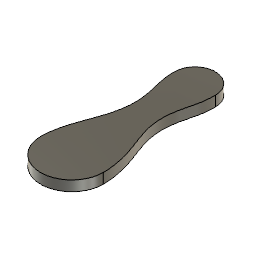
Linker (Autodesk Fusion 360 design; units mm, degrees)
part number: 2026-08-19-17-32-45-715
Autodesk Fusion 360 part; units mm, degrees
sketch "Sketch1" plane through (0, 0, 0) normal (0, 0, 1) x (1, 0, 0)
  circle A0 centre (0, 0) radius 30.539
  line L0 (0, 0) -> (0, 120)
  circle A1 centre (0, 120) radius 20
  spline S0 degree 5 poles (-20, 120) (-20, 118.6277) (-19.9377, 115.9337) (-19.6572, 112.0444) (-18.9403, 107.1368) (-17.656, 101.3217) (-16.2249, 95.6467) (-14.9004, 89.9411) (-13.9014, 84.0874) (-13.366, 78.0653) (-13.3647, 71.9193) (-13.9112, 65.7277) (-14.9727, 59.5726) (-16.479, 53.5086) (-18.3305, 47.5345) (-20.4074, 41.616) (-22.5782, 35.7039) (-24.7076, 29.7542) (-26.6645, 23.7473) (-28.3301, 17.7088) (-29.6027, 11.6919) (-30.2422, 6.9451) (-30.485, 3.446) (-30.539, 1.1436) (-30.539, 0) knots 0 0 0 0 0 0 0.05 0.1 0.15 0.2 0.25 0.3 0.35 0.4 0.45 0.5 0.55 0.6 0.65 0.7 0.75 0.8 0.85 0.9 0.95 1 1 1 1 1 1
  spline S1 degree 5 poles (30.539, 0) (30.539, 1.0785) (30.4943, 3.2756) (30.2934, 6.6915) (29.7578, 11.4626) (28.6529, 17.655) (27.1407, 23.9143) (25.276, 30.0944) (23.1495, 36.1084) (20.8974, 41.9731) (18.682, 47.7676) (16.6729, 53.5953) (15.0282, 59.5445) (13.8753, 65.6511) (13.2908, 71.8554) (13.2981, 78.0447) (13.8651, 84.101) (14.9009, 89.9465) (16.2511, 95.5906) (17.6914, 101.1783) (18.9706, 106.9311) (19.6763, 111.8544) (19.9473, 115.8136) (20.0032, 118.5829) (20, 120) knots 0 0 0 0 0 0 0.05 0.1 0.15 0.2 0.25 0.3 0.35 0.4 0.45 0.5 0.55 0.6 0.65 0.7 0.75 0.8 0.85 0.9 0.95 1 1 1 1 1 1
  line L1 (30.539, -11) -> (30.539, 11)
  line L2 (-30.539, 11.7182) -> (-30.539, -11.7182)
  line L3 (-20, 134) -> (-20, 106)
  line L4 (20.0327, 105.5399) -> (19.9673, 134.4601)
  point P0 (-30.539, 0)
  point P1 (30.539, 0)
  point P2 (-20, 120)
  point P3 (20, 120)
  point P4 (-24.7648, 29.445)
  point P5 (-15, 60)
  point P6 (-15, 90)
  point P7 (25.2479, 29.94)
  point P8 (15.0558, 60)
  point P9 (15, 90)
  point P10 (-15, 90)
  point P11 (-15, 60)
  point P12 (-24.7648, 29.445)
  point P13 (25.2479, 29.94)
  point P14 (15.0558, 60)
  point P15 (15, 90)
  dimension "d1" = 61.078
  dimension "d2" = 120
  dimension "d3" = 40
  constraint coincident A0.centre L0.start
  constraint vertical L0
  constraint coincident L0.end A1.centre
  constraint coincident A0 P0
  constraint coincident A0 P1
  constraint coincident A1 P2
  constraint coincident A1 P3
  constraint coincident P2 S0.start
  constraint coincident P10 P6
  constraint coincident P11 P5
  constraint coincident P12 P4
  constraint coincident P0 S0.end
  constraint coincident P1 S1.start
  constraint coincident P13 P7
  constraint coincident P14 P8
  constraint coincident P15 P9
  constraint coincident P3 S1.end
  constraint midpoint P1 L1
  constraint tangent A0 L1
  constraint midpoint P0 L2
  constraint tangent A0 L2
  constraint midpoint P2 L3
  constraint midpoint P3 L4
  measures "d1" diameter of A0
  measures "d2" distance of A0.centre L0.end
  measures "d3" diameter of A1
extrude "Extrude1" add sketch "Sketch1" along normal blind 10
sketch "Sketch2" plane through (0, 0, 0) normal (0, 0, 1) x (1, 0, 0)
sketch "Sketch3" plane through (0, 0, 0) normal (0, 0, -1) x (1, 0, 0)
  spline S0 degree 5 poles (30.539, 0) (30.539, -1.0785) (30.4943, -3.2756) (30.2934, -6.6915) (29.7578, -11.4626) (28.6529, -17.655) (27.1407, -23.9143) (25.276, -30.0944) (23.1495, -36.1084) (20.8974, -41.9731) (18.682, -47.7676) (16.6729, -53.5953) (15.0282, -59.5445) (13.8753, -65.6511) (13.2908, -71.8554) (13.2981, -78.0447) (13.8651, -84.101) (14.9009, -89.9465) (16.2511, -95.5906) (17.6914, -101.1783) (18.9706, -106.9311) (19.6763, -111.8544) (19.9473, -115.8136) (20.0032, -118.5829) (20, -120) knots 0 0 0 0 0 0 0.05 0.1 0.15 0.2 0.25 0.3 0.35 0.4 0.45 0.5 0.55 0.6 0.65 0.7 0.75 0.8 0.85 0.9 0.95 1 1 1 1 1 1
  arc A0 (30.539, 0) -> (-30.539, 0) centre (0, 0) ccw
  spline S1 degree 5 poles (-20, -120) (-20, -118.6277) (-19.9377, -115.9337) (-19.6572, -112.0444) (-18.9403, -107.1368) (-17.656, -101.3217) (-16.2249, -95.6467) (-14.9004, -89.9411) (-13.9014, -84.0874) (-13.366, -78.0653) (-13.3647, -71.9193) (-13.9112, -65.7277) (-14.9727, -59.5726) (-16.479, -53.5086) (-18.3305, -47.5345) (-20.4074, -41.616) (-22.5782, -35.7039) (-24.7076, -29.7542) (-26.6645, -23.7473) (-28.3301, -17.7088) (-29.6027, -11.6919) (-30.2422, -6.9451) (-30.485, -3.446) (-30.539, -1.1436) (-30.539, 0) knots 0 0 0 0 0 0 0.05 0.1 0.15 0.2 0.25 0.3 0.35 0.4 0.45 0.5 0.55 0.6 0.65 0.7 0.75 0.8 0.85 0.9 0.95 1 1 1 1 1 1
  arc A1 (-20, -120) -> (20, -120) centre (0, -120) ccw
  circle A2 centre (0, 0) radius 2.5
  circle A3 centre (0, -120) radius 2.5
  dimension "d6" = 5
  dimension "d7" = 5
  constraint coincident A0.centre A2.centre
  constraint concentric A1 A3
  measures "d6" diameter of A2
  measures "d7" diameter of A3
extrude "Extrude2" cut sketch "Sketch3" against normal blind 4 contours A2 | A3
